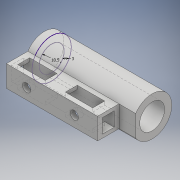
# Autodesk Inventor part: magnet-holder
Saved by Autodesk Inventor 2018 (Build 220112000, 112)
## iProperties
Created: 2025-02-27
Part Number: magnet-holder
Material: Generic
Document SubType Name: Modeling
Designer: neo
Density: 1 g/cm^3
Appearance: Default
Author: neo
Autodesk Inventor part; units mm, degrees
ref_plane "YZ Plane" through (0, 0, 0) normal (1, 0, 0) x (0, 1, 0)
ref_plane "XZ Plane" through (0, 0, 0) normal (0, 1, 0) x (-1, 0, 0)
ref_plane "XY Plane" through (0, 0, 0) normal (0, 0, 1) x (1, 0, 0)
sketch "Sketch1" plane through (0, 0, 0) normal (1, 0, 0) x (0, 1, 0)
  circle A0 centre (0, 0) radius 5.25
  circle A1 centre (0, 0) radius 8.25
  dimension "d0" = 10.5
  dimension "d1" = 3
  constraints: 2 centre point, 2 coincident
  measures "d0" diameter of A0
  measures "d1" radial gap between concentric circles of A0 A1
extrude "Extrusion1" add sketch "Sketch1" along normal blind 42.3
extrude "Extrusion2" add sketch "Sketch1" against normal blind 3 contours A0 | A1
sketch "Sketch2" plane through (-3, 0, 0) normal (-1, 0, 0) x (0, 0, 1)
  circle A0 centre (0, 0) radius 8.25 projected
  line L0 (0, 0) -> (0, -27.9762)
  line L1 (-4.5, -6.9147) -> (4.5, -6.9147)
  line L2 (4.5, -6.9147) -> (4.5, -15.9147)
  line L3 (4.5, -15.9147) -> (-4.5, -15.9147)
  line L4 (-4.5, -15.9147) -> (-4.5, -6.9147)
  line L5 (-3, -8.9147) -> (3, -8.9147)
  line L6 (3, -8.9147) -> (3, -13.9147)
  line L7 (3, -13.9147) -> (-3, -13.9147)
  line L8 (-3, -13.9147) -> (-3, -8.9147)
  dimension "d6" = 9
  dimension "d7" = 2
  dimension "d8" = 6
  dimension "d9" = 2
  dimension "d10" = 5
  constraints: 18 end point, 4 parallel, 2 horizontal, 2 perpendicular, 1 vertical, 4 other
  measures "d6" distance of L2.end L3.end
  measures "d7" distance between parallel lines of L3 L7
  measures "d8" distance between parallel lines of L8 L6
  measures "d9" distance between parallel lines of L5 L1
  measures "d10" distance of L5.end L6.end
extrude "Extrusion3" add sketch "Sketch2" against normal up to surface (45.3 mm away) contours L1 L0 A0 | A0 L0 L5 L8 L7 L3 L4 | L2 L3 L0 L7 L6 L5 A0 | A0 L0 L1
sketch "Sketch3" plane through (-3, -15.9147, -4.5) normal (0, -1, 0) x (1, 0, 0)
  line L0 (45.3, 0) -> (45.3, 9) projected
  line L1 (0, 9) -> (45.3, 9) projected
  line L2 (0, 9) -> (0, 0) construction
  line L3 (0, 0) -> (45.3, 0) projected
  line L4 (0, 12.75) -> (0, -3.75) construction
  line L5 (0, 4.5) -> (45.3, 4.5)
  circle A0 centre (8.5, 4.5) radius 1.75
  circle A1 centre (28.5, 4.5) radius 1.75
  point P0 (3, 4.5)
  dimension "d13" = 3.5
  dimension "d16" = 20
  dimension "d21" = 8.5
  constraints: 2 centre point, 2 end point, 2 midpoint, 1 horizontal, 1 point on line, 2 other
  measures "d13" diameter of A0
  measures "d16" distance of A0.centre A1.centre
  measures "d21" distance from line of L2 A0.centre
extrude "Extrusion4" cut sketch "Sketch3" against normal up to surface (2 mm away)
ref_plane "Work Plane1" through (5.5, -15.9147, 1.75) normal (0, 0, 1) x (1, 0, 0)
sketch "Sketch4" plane through (5.5, -15.9147, 1.75) normal (0, 0, 1) x (1, 0, 0)
  line L0 (-1.75, 0) -> (-1.75, 2) projected
  line L1 (1.75, 0) -> (1.75, 2) projected
  line L2 (18.25, 0) -> (18.25, 2) projected
  line L3 (21.75, 0) -> (21.75, 2) projected
  line L4 (-8.5, 7) -> (36.8, 7) projected
  line L5 (-8.5, 2) -> (36.8, 2) projected
  line L6 (-5.75, 7) -> (5.75, 7)
  line L7 (5.75, 7) -> (5.75, 2)
  line L8 (5.75, 2) -> (-5.75, 2)
  line L9 (-5.75, 2) -> (-5.75, 7)
  line L10 (14.25, 7) -> (25.75, 7)
  line L11 (25.75, 7) -> (25.75, 2)
  line L12 (25.75, 2) -> (14.25, 2)
  line L13 (14.25, 2) -> (14.25, 7)
  point P0 (-5.5, 15.9147)
  dimension "d24" = 4
  dimension "d25" = 4
  dimension "d26" = 4
  dimension "d27" = 4
  constraints: 16 end point, 4 parallel, 4 point on line, 2 horizontal, 2 perpendicular
  measures "d24" distance between parallel lines of L9 L0
  measures "d25" distance between parallel lines of L1 L7
  measures "d26" distance between parallel lines of L13 L2
  measures "d27" distance between parallel lines of L3 L11
extrude "Extrusion5" cut sketch "Sketch4" along normal through all both and the other way through all contours L4 L7 L5 L9 | L4 L11 L5 L13
sketch "Sketch5" plane through (-3, -15.9147, 4.5) normal (0, 0, 1) x (1, 0, 0)
  line L0 (14.25, 2) -> (2.75, 2) projected
  line L1 (2.75, 2) -> (2.75, 7) projected
  line L2 (2.75, 7) -> (14.25, 7) projected
  line L3 (14.25, 7) -> (14.25, 2) projected
  line L4 (34.25, 2) -> (22.75, 2) projected
  line L5 (22.75, 2) -> (22.75, 7) projected
  line L6 (22.75, 7) -> (34.25, 7) projected
  line L7 (34.25, 7) -> (34.25, 2) projected
  line L8 (45.3, 0) -> (45.3, 9) projected
  line L9 (0, 9) -> (45.3, 9) projected
  line L10 (0, 9) -> (0, 0) projected
  line L11 (0, 0) -> (45.3, 0) projected
  line L12 (0, 9) -> (45.3, 9) projected
  line L13 (0, 0) -> (45.3, 0) projected
  line L14 (45.3, 9) -> (38.3, 9)
  line L15 (38.3, 9) -> (38.3, 0)
  line L16 (38.3, 0) -> (45.3, 0)
  line L17 (45.3, 0) -> (45.3, 9)
  point P0 (3, 15.9147)
  dimension "d30" = 7
  constraints: 8 end point, 2 parallel, 1 horizontal, 1 perpendicular, 1 point on line
  measures "d30" distance between parallel lines of L8 L15
extrude "Extrusion6" cut sketch "Sketch5" against normal through all contours L11 L15 L9 L8
body "Solid1"
